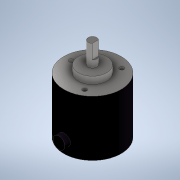
# Autodesk Inventor part: E6B2-CWZ6C
Saved by Autodesk Inventor 2020 (Build 240168000, 168)
## iProperties
Created: 2021-06-11
Part Number: E6B2-CWZ6C
Material: 一般
Document SubType Name: Modeling
Designer: user
Density: 1 g/cm^3
Appearance: 鍍鋅
Author: user
Autodesk Inventor part; units mm, degrees
ref_plane "YZ Plane" through (0, 0, 0) normal (1, 0, 0) x (0, 1, 0)
ref_plane "XZ Plane" through (0, 0, 0) normal (0, 1, 0) x (-1, 0, 0)
sketch "草圖1" plane through (0, 0, 0) normal (0, 1, 0) x (-1, 0, 0)
  circle A0 centre (0, 0) radius 20.055
  dimension "d0" = 40.11
  constraints: 1 centre point, 1 coincident
  measures "d0" diameter of A0
extrude "擠出1" add sketch "草圖1" along normal blind 39
sketch "草圖2" plane through (0, 39, 0) normal (0, 1, 0) x (1, 0, 0)
  circle A0 centre (0, 0) radius 9.94
  dimension "d3" = 19.88
  constraints: 1 centre point, 1 coincident
  measures "d3" diameter of A0
extrude "擠出2" add sketch "草圖2" along normal blind 5
sketch "草圖3" plane through (0, 44, 0) normal (0, 1, 0) x (1, 0, 0)
  circle A0 centre (0, 0) radius 3
  dimension "d6" = 6
  constraints: 1 centre point, 1 coincident
  measures "d6" diameter of A0
extrude "擠出3" add sketch "草圖3" along normal blind 15
sketch "草圖4" plane through (0, 59, 0) normal (0, 1, 0) x (1, 0, 0)
  circle A0 centre (0, 0) radius 3 projected
  line L0 (-16.4783, -20) -> (15.8218, -20) construction
  line L1 (2, 2.2361) -> (2, -2.2361)
  arc A1 (2, -2.2361) -> (2, 2.2361) centre (0, 0) ccw
  point P0 (-3, 0)
  dimension "d9" = 20
  dimension "d10" = 20
  dimension "d11" = 5
  constraints: 4 end point, 2 point on circle, 1 centre point, 1 coincident, 1 horizontal, 1 vertical, 3 other
  measures "d9" distance from line of point (0, 0) L0
  measures "d10" distance from line of L0 point (-3, 0)
  measures "d11" distance from line of point (-3, 0) L1
extrude "擠出4" cut sketch "草圖4" against normal blind 10 contours A0 L1 picked at (2.1409, -0.5898)
ref_plane "工作平面2" through (0, 0, 20) normal (0, 0, 1) x (1, 0, 0)
sketch "草圖5" plane through (0, 0, 20) normal (0, 0, 1) x (1, 0, 0)
  circle A0 centre (0, 8.45) radius 4.15
  point P0 (0, 0)
  dimension "d16" = 8.3
  dimension "d17" = 8.45
  constraints: 1 centre point
  measures "d16" diameter of A0
  measures "d17" distance of point (0, 0) A0.centre
extrude "擠出5" add sketch "草圖5" along normal mid plane 7.11
sketch "草圖6" plane through (0, 39, 0) normal (0, 1, 0) x (1, 0, 0)
  circle A0 centre (-15, 0) radius 1.5
  circle A1 centre (7.5, -12.9904) radius 1.5
  circle A2 centre (7.5, 12.9904) radius 1.5
  line L0 (0, 0) -> (7.5, -12.9904) construction
  arc A3 (2, 2.2361) -> (2, -2.2361) centre (0, 0) ccw projected
  line L1 (0, 0) -> (7.5, 12.9904) construction
  line L2 (0, 0) -> (-20.055, 0) construction
  circle A4 centre (0, 0) radius 20.055 projected
  dimension "d20" = 120
  dimension "d21" = 120
  dimension "d22" = 3
  dimension "d23" = 15
  dimension "d24" = 15
  dimension "d25" = 15
  constraints: 8 end point, 3 centre point, 2 equal radius, 1 horizontal, 1 horizontal alignment, 1 point on line, 1 other
  measures "d20" angle of L0 L2
  measures "d21" angle of L2 L1
  measures "d22" diameter of A0
  measures "d23" distance of L0.start A0.centre
  measures "d24" distance of L0.start L0.end
  measures "d25" distance of L1.start L1.end
extrude "擠出6" cut sketch "草圖6" against normal blind 7 contours A0 | A1 | A2
